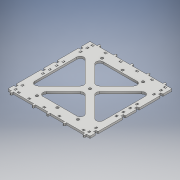
# Autodesk Inventor part: turtlebot_installation_side
Saved by Autodesk Inventor 2018 (Build 220112000, 112)
## iProperties
Created: 2018-07-15
Part Number: turtlebot_installation_side
Material: Generic
Document SubType Name: Modeling
Designer: Tsche
Density: 1 g/cm^3
Appearance: Default
Author: Tsche
Autodesk Inventor part; units mm, degrees
ref_plane "YZ Plane" through (0, 0, 0) normal (1, 0, 0) x (0, 1, 0)
ref_plane "XZ Plane" through (0, 0, 0) normal (0, 1, 0) x (-1, 0, 0)
ref_plane "XY Plane" through (0, 0, 0) normal (0, 0, 1) x (1, 0, 0)
sketch "Sketch1" plane through (0, 0, 0) normal (0, 0, 1) x (1, 0, 0)
  line L0 (-60, 60) -> (-49.5, 60)
  line L1 (60, 60) -> (60, 46.6)
  line L2 (60, -60) -> (55, -60)
  line L3 (-60, -60) -> (-60, -51.6)
  line L4 (-60, 60) -> (60, -60) construction
  line L5 (60, 60) -> (-60, -60) construction
  line L6 (-52, -60) -> (-52, -63)
  line L7 (-52, -63) -> (-55, -63)
  line L8 (-55, -63) -> (-55, -60)
  line L9 (-19.5, -60) -> (-19.5, -63)
  line L10 (-19.5, -63) -> (-22.5, -63)
  line L11 (-22.5, -63) -> (-22.5, -60)
  line L12 (-55, -60) -> (-60, -60)
  line L13 (-52, -60) -> (-55, -60) construction
  line L14 (-22.5, -60) -> (-52, -60)
  line L15 (-19.5, -60) -> (-22.5, -60) construction
  line L16 (-1.5, -60) -> (-19.5, -60)
  line L17 (22.75, -60) -> (1.5, -60)
  line L18 (52, -60) -> (25.75, -60)
  line L19 (-21, -63) -> (-21, -60) construction
  line L20 (-53.5, -60) -> (-53.5, -63) construction
  line L21 (-49, -55.7) -> (-46, -55.7)
  line L22 (-46, -55.7) -> (-46, -57)
  line L23 (-46, -57) -> (-49, -57)
  line L24 (-49, -57) -> (-49, -55.7)
  line L25 (-47.5, -57) -> (-47.5, -55.7) construction
  line L26 (-33.5, -55.7) -> (-30.5, -55.7)
  line L27 (-30.5, -55.7) -> (-30.5, -57)
  line L28 (-30.5, -57) -> (-33.5, -57)
  line L29 (-33.5, -57) -> (-33.5, -55.7)
  line L30 (-32, -57) -> (-32, -55.7) construction
  line L31 (0, -7.0711) -> (-36.9289, -44)
  line L32 (36.9289, -44) -> (0, -7.0711)
  line L33 (-84, 0) -> (84, 0) construction
  line L34 (0, 7.0711) -> (-36.9289, 44)
  line L35 (36.9289, 44) -> (0, 7.0711)
  line L36 (-7.0711, 0) -> (-50, -42.9289)
  line L37 (-50, -42.9289) -> (-50, 42.9289)
  line L38 (-50, 42.9289) -> (-7.0711, 0)
  line L39 (7.0711, 0) -> (50, -42.9289)
  line L40 (50, -42.9289) -> (50, 42.9289)
  line L41 (50, 42.9289) -> (7.0711, 0)
  line L42 (-60, -48.4) -> (-60, -11.6)
  line L43 (-60, 11.6) -> (-60, 43.4)
  line L44 (60, -51.6) -> (60, -60)
  line L45 (60, 8.4) -> (60, -8.4)
  line L46 (-54, -43.5) -> (-52.7, -43.5)
  line L47 (-52.7, -43.5) -> (-52.7, -46.5)
  line L48 (-52.7, -46.5) -> (-54, -46.5)
  line L49 (-54, -46.5) -> (-54, -43.5)
  line L50 (-54, 6.5) -> (-52.7, 6.5)
  line L51 (-52.7, 6.5) -> (-52.7, 3.5)
  line L52 (-52.7, 3.5) -> (-54, 3.5)
  line L53 (-54, 3.5) -> (-54, 6.5)
  line L54 (-54, 16.5) -> (-52.7, 16.5)
  line L55 (-52.7, 16.5) -> (-52.7, 13.5)
  line L56 (-52.7, 13.5) -> (-54, 13.5)
  line L57 (-54, 13.5) -> (-54, 16.5)
  line L58 (52.7, 16.5) -> (54, 16.5)
  line L59 (54, 16.5) -> (54, 13.5)
  line L60 (54, 13.5) -> (52.7, 13.5)
  line L61 (52.7, 13.5) -> (52.7, 16.5)
  line L62 (52.7, 6.5) -> (54, 6.5)
  line L63 (54, 6.5) -> (54, 3.5)
  line L64 (54, 3.5) -> (52.7, 3.5)
  line L65 (52.7, 3.5) -> (52.7, 6.5)
  line L66 (52.7, -43.5) -> (54, -43.5)
  line L67 (54, -43.5) -> (54, -46.5)
  line L68 (54, -46.5) -> (52.7, -46.5)
  line L69 (52.7, -46.5) -> (52.7, -43.5)
  line L70 (-54, -45) -> (-52.7, -45) construction
  line L71 (-54, 5) -> (-52.7, 5) construction
  line L72 (-54, 15) -> (-52.7, 15) construction
  line L73 (52.7, 15) -> (54, 15) construction
  line L74 (52.7, 5) -> (54, 5) construction
  line L75 (52.7, -45) -> (54, -45) construction
  line L76 (0, 60) -> (0, -60) construction
  line L77 (0, 88.2) -> (0, -88.2) construction
  line L78 (-1.5, -60) -> (1.5, -60) construction
  line L79 (22.75, -60) -> (25.75, -60) construction
  line L80 (52, -60) -> (55, -60) construction
  line L81 (60, -51.6) -> (60, -48.4) construction
  line L82 (60, 11.6) -> (60, 8.4) construction
  line L83 (-60, 8.4) -> (-60, 11.6) construction
  line L84 (-60, -48.4) -> (-60, -51.6) construction
  line L85 (60, 11.6) -> (56.9, 11.6)
  line L86 (56.9, 11.6) -> (56.9, 8.4)
  line L87 (56.9, 8.4) -> (60, 8.4)
  line L88 (60, -48.4) -> (56.9, -48.4)
  line L89 (56.9, -48.4) -> (56.9, -51.6)
  line L90 (56.9, -51.6) -> (60, -51.6)
  line L91 (56.9, -50) -> (60, -50) construction
  line L92 (56.9, 10) -> (60, 10) construction
  line L93 (-60, -48.4) -> (-56.9, -48.4)
  line L94 (-56.9, -48.4) -> (-56.9, -51.6)
  line L95 (-56.9, -51.6) -> (-60, -51.6)
  line L96 (-60, -50) -> (-56.9, -50) construction
  line L97 (-60, 11.6) -> (-56.9, 11.6)
  line L98 (-56.9, 11.6) -> (-56.9, 8.4)
  line L99 (-56.9, 8.4) -> (-60, 8.4)
  line L100 (-60, 10) -> (-56.9, 10) construction
  line L101 (-1.5, -60) -> (-1.5, -63)
  line L102 (-1.5, -63) -> (1.5, -63)
  line L103 (1.5, -63) -> (1.5, -60)
  line L104 (22.75, -60) -> (22.75, -63)
  line L105 (22.75, -63) -> (25.75, -63)
  line L106 (25.75, -63) -> (25.75, -60)
  line L107 (52, -60) -> (52, -63)
  line L108 (52, -63) -> (55, -63)
  line L109 (55, -63) -> (55, -60)
  line L110 (53.5, -60) -> (53.5, -63) construction
  line L111 (24.25, -60) -> (24.25, -63) construction
  line L112 (-11.5, -55.7) -> (-8.5, -55.7)
  line L113 (-8.5, -55.7) -> (-8.5, -57)
  line L114 (-8.5, -57) -> (-11.5, -57)
  line L115 (-11.5, -57) -> (-11.5, -55.7)
  line L116 (-10, -55.7) -> (-10, -57) construction
  line L117 (10.625, -55.7) -> (13.625, -55.7)
  line L118 (13.625, -55.7) -> (13.625, -57)
  line L119 (13.625, -57) -> (10.625, -57)
  line L120 (10.625, -57) -> (10.625, -55.7)
  line L121 (12.125, -55.7) -> (12.125, -57) construction
  line L122 (46, -55.7) -> (49, -55.7)
  line L123 (49, -55.7) -> (49, -57)
  line L124 (49, -57) -> (46, -57)
  line L125 (46, -57) -> (46, -55.7)
  line L126 (47.5, -55.7) -> (47.5, -57) construction
  line L127 (-1.5, 60) -> (-1.5, 63)
  line L128 (-1.5, 63) -> (1.5, 63)
  line L129 (1.5, 63) -> (1.5, 60)
  line L130 (-1.5, 60) -> (1.5, 60) construction
  line L131 (1.5, 60) -> (22.5, 60)
  line L132 (-22.5, 60) -> (-22.5, 63)
  line L133 (-22.5, 63) -> (-25.5, 63)
  line L134 (-25.5, 63) -> (-25.5, 60)
  line L135 (-46.5, 60) -> (-46.5, 63)
  line L136 (-46.5, 63) -> (-49.5, 63)
  line L137 (-49.5, 63) -> (-49.5, 60)
  line L138 (22.5, 60) -> (22.5, 63)
  line L139 (22.5, 63) -> (25.5, 63)
  line L140 (25.5, 63) -> (25.5, 60)
  line L141 (46.5, 60) -> (46.5, 63)
  line L142 (46.5, 63) -> (49.5, 63)
  line L143 (49.5, 63) -> (49.5, 60)
  line L144 (-49.5, 60) -> (-46.5, 60) construction
  line L145 (-46.5, 60) -> (-25.5, 60)
  line L146 (-25.5, 60) -> (-22.5, 60) construction
  line L147 (-22.5, 60) -> (-1.5, 60)
  line L148 (22.5, 60) -> (25.5, 60) construction
  line L149 (25.5, 60) -> (46.5, 60)
  line L150 (46.5, 60) -> (49.5, 60) construction
  line L151 (49.5, 60) -> (60, 60)
  line L152 (-48, 63) -> (-48, 60) construction
  line L153 (-24, 63) -> (-24, 60) construction
  line L154 (24, 63) -> (24, 60) construction
  line L155 (48, 63) -> (48, 60) construction
  line L156 (-13.5, 57) -> (-10.5, 57)
  line L157 (-10.5, 57) -> (-10.5, 55.7)
  line L158 (-10.5, 55.7) -> (-13.5, 55.7)
  line L159 (-13.5, 55.7) -> (-13.5, 57)
  line L160 (-12, 57) -> (-12, 55.7) construction
  line L161 (-32.5, 57) -> (-32.5, 55.7)
  line L162 (-34, 57) -> (-34, 55.7) construction
  line L163 (-35.5, 57) -> (-32.5, 57)
  line L164 (-35.5, 55.7) -> (-35.5, 57)
  line L165 (-32.5, 55.7) -> (-35.5, 55.7)
  line L166 (-54.5, 55.7) -> (-54.5, 57)
  line L167 (-53, 57) -> (-53, 55.7) construction
  line L168 (-51.5, 57) -> (-51.5, 55.7)
  line L169 (-54.5, 57) -> (-51.5, 57)
  line L170 (-51.5, 55.7) -> (-54.5, 55.7)
  line L171 (13.5, 57) -> (10.5, 57)
  line L172 (10.5, 57) -> (10.5, 55.7)
  line L173 (10.5, 55.7) -> (13.5, 55.7)
  line L174 (13.5, 55.7) -> (13.5, 57)
  line L175 (12, 57) -> (12, 55.7) construction
  line L176 (32.5, 57) -> (32.5, 55.7)
  line L177 (34, 57) -> (34, 55.7) construction
  line L178 (35.5, 57) -> (32.5, 57)
  line L179 (35.5, 55.7) -> (35.5, 57)
  line L180 (32.5, 55.7) -> (35.5, 55.7)
  line L181 (54.5, 55.7) -> (54.5, 57)
  line L182 (53, 57) -> (53, 55.7) construction
  line L183 (51.5, 57) -> (51.5, 55.7)
  line L184 (54.5, 57) -> (51.5, 57)
  line L185 (51.5, 55.7) -> (54.5, 55.7)
  line L186 (-54, -56.5) -> (-52.7, -56.5)
  line L187 (-52.7, -56.5) -> (-52.7, -53.5)
  line L188 (-52.7, -53.5) -> (-54, -53.5)
  line L189 (-54, -53.5) -> (-54, -56.5)
  line L190 (-54, -55) -> (-52.7, -55) construction
  line L191 (52.7, -56.5) -> (54, -56.5)
  line L192 (54, -56.5) -> (54, -53.5)
  line L193 (54, -53.5) -> (52.7, -53.5)
  line L194 (52.7, -53.5) -> (52.7, -56.5)
  line L195 (52.7, -55) -> (54, -55) construction
  line L196 (-60, -8.4) -> (-56.9, -8.4)
  line L197 (-56.9, -8.4) -> (-56.9, -11.6)
  line L198 (-56.9, -11.6) -> (-60, -11.6)
  line L199 (-60, -8.4) -> (-60, 8.4)
  line L200 (-60, -11.6) -> (-60, -8.4) construction
  line L201 (-60, -10) -> (-56.9, -10) construction
  line L202 (-54, -3.5) -> (-52.7, -3.5)
  line L203 (-52.7, -3.5) -> (-52.7, -6.5)
  line L204 (-52.7, -6.5) -> (-54, -6.5)
  line L205 (-54, -6.5) -> (-54, -3.5)
  line L206 (-54, -5) -> (-52.7, -5) construction
  line L207 (-54, -16.5) -> (-52.7, -16.5)
  line L208 (-52.7, -16.5) -> (-52.7, -13.5)
  line L209 (-52.7, -13.5) -> (-54, -13.5)
  line L210 (-54, -13.5) -> (-54, -16.5)
  line L211 (-54, -15) -> (-52.7, -15) construction
  line L212 (60, -8.4) -> (56.9, -8.4)
  line L213 (56.9, -8.4) -> (56.9, -11.6)
  line L214 (56.9, -11.6) -> (60, -11.6)
  line L215 (60, -8.4) -> (60, -11.6) construction
  line L216 (60, -10) -> (56.9, -10) construction
  line L217 (60, -11.6) -> (60, -48.4)
  line L218 (54, -3.5) -> (52.7, -3.5)
  line L219 (52.7, -3.5) -> (52.7, -6.5)
  line L220 (52.7, -6.5) -> (54, -6.5)
  line L221 (54, -6.5) -> (54, -3.5)
  line L222 (54, -5) -> (52.7, -5) construction
  line L223 (54, -15) -> (52.7, -15) construction
  line L224 (54, -16.5) -> (52.7, -16.5)
  line L225 (52.7, -16.5) -> (52.7, -13.5)
  line L226 (54, -13.5) -> (54, -16.5)
  line L227 (52.7, -13.5) -> (54, -13.5)
  line L228 (-60, 46.6) -> (-56.9, 46.6)
  line L229 (-56.9, 46.6) -> (-56.9, 43.4)
  line L230 (-56.9, 43.4) -> (-60, 43.4)
  line L231 (-60, 46.6) -> (-60, 60)
  line L232 (-60, 43.4) -> (-60, 46.6) construction
  line L233 (-60, 45) -> (-56.9, 45) construction
  line L234 (-54, 41.5) -> (-52.7, 41.5)
  line L235 (-52.7, 41.5) -> (-52.7, 38.5)
  line L236 (-52.7, 38.5) -> (-54, 38.5)
  line L237 (-54, 38.5) -> (-54, 41.5)
  line L238 (-54, 40) -> (-52.7, 40) construction
  line L239 (-54, 48.5) -> (-52.7, 48.5)
  line L240 (-52.7, 48.5) -> (-52.7, 51.5)
  line L241 (-52.7, 51.5) -> (-54, 51.5)
  line L242 (-54, 51.5) -> (-54, 48.5)
  line L243 (-54, 50) -> (-52.7, 50) construction
  line L244 (60, 46.6) -> (56.9, 46.6)
  line L245 (56.9, 46.6) -> (56.9, 43.4)
  line L246 (56.9, 43.4) -> (60, 43.4)
  line L247 (60, 46.6) -> (60, 43.4) construction
  line L248 (60, 43.4) -> (60, 11.6)
  line L249 (56.9, 45) -> (60, 45) construction
  line L250 (54, 41.5) -> (52.7, 41.5)
  line L251 (52.7, 41.5) -> (52.7, 38.5)
  line L252 (52.7, 38.5) -> (54, 38.5)
  line L253 (54, 38.5) -> (54, 41.5)
  line L254 (54, 40) -> (52.7, 40) construction
  line L255 (54, 48.5) -> (52.7, 48.5)
  line L256 (54, 50) -> (52.7, 50) construction
  line L257 (54, 51.5) -> (54, 48.5)
  line L258 (52.7, 51.5) -> (54, 51.5)
  line L259 (52.7, 48.5) -> (52.7, 51.5)
  circle A0 centre (0, 47.625) radius 1.85
  circle A1 centre (0, -47.625) radius 1.85
  line L260 (36.9289, -44) -> (-36.9289, -44)
  line L261 (36.9289, 44) -> (-36.9289, 44)
  circle A2 centre (30, -47.625) radius 1.85
  circle A3 centre (-30, -47.625) radius 1.85
  circle A4 centre (30, 47.625) radius 1.85
  circle A5 centre (-30, 47.625) radius 1.85
  circle A6 centre (0, 0) radius 1.85
  point P0 (0, 0)
  point P1 (0, 0)
  point P2 (0, -63)
  point P3 (0, 63)
  point P4 (-31, 50)
  dimension "d0" = 120
  dimension "d1" = 120
  dimension "d2" = 3
  dimension "d3" = 3
  dimension "d12" = 3
  dimension "d13" = 3
  dimension "d15" = 6.5
  dimension "d19" = 32.5
  dimension "d20" = 3
  dimension "d21" = 1.3
  dimension "d28" = 6
  dimension "d30" = 3
  dimension "d31" = 1.3
  dimension "d32" = 11
  dimension "d35" = 3
  dimension "d36" = 10
  dimension "d37" = 5
  dimension "d38" = 5
  dimension "d51" = 3
  dimension "d52" = 1.3
  dimension "d53" = 3
  dimension "d54" = 3
  dimension "d55" = 1.3
  dimension "d56" = 1.3
  dimension "d57" = 3
  dimension "d58" = 1.3
  dimension "d59" = 3
  dimension "d60" = 3
  dimension "d61" = 1.3
  dimension "d85" = 60
  dimension "d86" = 10
  dimension "d87" = 3.2
  dimension "d88" = 3.2
  dimension "d90" = 3.1
  dimension "d92" = 3.1
  dimension "d93" = 3.2
  dimension "d94" = 10
  dimension "d95" = 3.1
  dimension "d96" = 3.2
  dimension "d97" = 60
  dimension "d98" = 5
  dimension "d99" = 6
  dimension "d100" = 5
  dimension "d101" = 6
  dimension "d102" = 5
  dimension "d103" = 5
  dimension "d104" = 6
  dimension "d105" = 5
  dimension "d106" = 3
  dimension "d107" = 3
  dimension "d108" = 3
  dimension "d109" = 6.5
  dimension "d110" = 24.25
  dimension "d111" = 3
  dimension "d112" = 1.3
  dimension "d113" = 3
  dimension "d114" = 1.3
  dimension "d115" = 3
  dimension "d116" = 1.3
  dimension "d117" = 12.125
  dimension "d118" = 6
  dimension "d119" = 11
  dimension "d122" = 3
  dimension "d123" = 3
  constraints: 520 end point, 174 parallel, 167 perpendicular, 76 symmetric about line, 69 midpoint, 41 point on line, 38 horizontal, 19 collinear, 13 equal length, 7 centre point, 7 vertical, 1 coincident, 1 equal radius, 29 other
  measures "d0" distance of L2.start L3.start
  measures "d1" distance of L1.start L2.start
  measures "d2" distance of L6.end L7.end
  measures "d3" distance of L6.start L6.end
  measures "d12" distance of L9.end L10.end
  measures "d13" distance of L9.start L9.end
  measures "d15" distance between parallel lines of L3 L20
  measures "d19" distance between parallel lines of L19 L20
  measures "d20" distance of L21.start L21.end
  measures "d21" distance of L23.end L21.start
  measures "d28" distance between parallel lines of L20 L25
  measures "d30" distance of L29.end L27.start
  measures "d31" distance of L29.start L29.end
  measures "d32" distance between parallel lines of L30 L19
  measures "d35" distance between parallel lines of L23 L14
  measures "d36" distance between parallel lines of L3 L37
  measures "d37" distance between parallel lines of L36 L5
  measures "d38" distance between parallel lines of L31 L5
  measures "d51" distance of L46.end L47.end
  measures "d52" distance of L47.end L48.end
  measures "d53" distance of L50.end L51.end
  measures "d54" distance of L54.end L55.end
  measures "d55" distance of L54.start L54.end
  measures "d56" distance of L58.start L58.end
  measures "d57" distance of L60.end L58.start
  measures "d58" distance of L63.end L64.end
  measures "d59" distance of L64.end L62.start
  measures "d60" distance of L68.end L66.start
  measures "d61" distance of L66.start L66.end
  measures "d85" distance between parallel lines of L92 L91
  measures "d86" distance between parallel lines of L2 L91
  measures "d87" distance of L85.end L86.end
  measures "d88" distance of L88.end L89.end
  measures "d90" distance of L86.end L45.start
  measures "d92" distance of L94.end L3.end
  measures "d93" distance of L93.end L94.end
  measures "d94" distance between parallel lines of L12 L96
  measures "d95" distance of L98.end L83.start
  measures "d96" distance of L97.end L98.end
  measures "d97" distance between parallel lines of L96 L100
  measures "d98" distance between parallel lines of L70 L96
  measures "d99" distance between parallel lines of L42 L49
  measures "d100" distance between parallel lines of L100 L71
  measures "d101" distance between parallel lines of L42 L53
  measures "d102" distance between parallel lines of L100 L72
  measures "d103" distance between parallel lines of L92 L73
  measures "d104" distance between parallel lines of L45 L63
  measures "d105" distance between parallel lines of L91 L75
  measures "d106" distance of L101.end L102.end
  measures "d107" distance of L104.end L105.end
  measures "d108" distance of L107.end L108.end
  measures "d109" distance between parallel lines of L44 L110
  measures "d110" distance between parallel lines of L77 L111
  measures "d111" distance of L113.end L114.end
  measures "d112" distance of L114.end L112.start
  measures "d113" distance of L119.start L120.start
  measures "d114" distance of L120.start L120.end
  measures "d115" distance of L124.start L125.start
  measures "d116" distance of L125.start L125.end
  measures "d117" distance between parallel lines of L77 L121
  measures "d118" distance between parallel lines of L110 L126
  measures "d119" distance between parallel lines of L19 L116
  measures "d122" distance of L127.end L128.end
  measures "d123" distance of L127.start L127.end
extrude "Extrusion2" add sketch "Sketch1" along normal blind 3
fillet "Fillet1" radius 1 40 edges at (-60, 11.6, 1.5) (-60, 8.4, 1.5) (-60, -60, 1.5) (-60, -51.6, 1.5) (-60, -48.4, 1.5) (-55, -63, 1.5) (-52, -63, 1.5) (-22.5, -63, 1.5) (-19.5, -63, 1.5) (-1.5, -63, 1.5) (1.5, -63, 1.5) (22.75, -63, 1.5) (25.75, -63, 1.5) (52, -63, 1.5) (55, -63, 1.5) (60, -60, 1.5) (60, -51.6, 1.5) (60, -48.4, 1.5) (60, 8.4, 1.5) (60, 11.6, 1.5) (-49.5, 63, 1.5) (-46.5, 63, 1.5) (-60, 60, 1.5) (-25.5, 63, 1.5) (-22.5, 63, 1.5) (-1.5, 63, 1.5) (1.5, 63, 1.5) (22.5, 63, 1.5) (25.5, 63, 1.5) (46.5, 63, 1.5) (49.5, 63, 1.5) (60, 60, 1.5) (-60, -11.6, 1.5) (-60, -8.4, 1.5) (60, -11.6, 1.5) (60, -8.4, 1.5) (-60, 43.4, 1.5) (-60, 46.6, 1.5) (60, 43.4, 1.5) (60, 46.6, 1.5)
chamfer "Chamfer1" distance 1 angle 45 54 edges at (-54, 15, 3) (-54, 15, 0) (-54, 5, 3) (-54, 5, 0) (-54, -45, 3) (-54, -45, 0) (-47.5, -57, 3) (-47.5, -57, 0) (-32, -57, 3) (-32, -57, 0) (-10, -57, 3) (-10, -57, 0) (12.125, -57, 3) (12.125, -57, 0) (47.5, -57, 3) (47.5, -57, 0) (54, -45, 3) (54, -45, 0) (54, 5, 3) (54, 5, 0) (54, 15, 3) (54, 15, 0) (-53, 57, 3) (-53, 57, 0) (-34, 57, 3) (-34, 57, 0) (-12, 57, 3) (-12, 57, 0) (12, 57, 3) (12, 57, 0) (34, 57, 3) (34, 57, 0) (53, 57, 3) (53, 57, 0) (-54, -55, 3) (-54, -55, 0) (54, -55, 0) (54, -55, 3) (-54, -5, 3) (-54, -15, 3) (-54, -5, 0) (-54, -15, 0) (54, -15, 3) (54, -15, 0) (54, -5, 3) (54, -5, 0) (54, 40, 0) (54, 40, 3) (54, 50, 0) (54, 50, 3) (-54, 40, 3) (-54, 40, 0) (-54, 50, 0) (-54, 50, 3)
fillet "Fillet2" radius 5 12 edges at (-50, 42.9289, 1.5) (-36.9289, 44, 1.5) (36.9289, 44, 1.5) (0, 7.0711, 1.5) (-7.0711, 0, 1.5) (7.0711, 0, 1.5) (0, -7.0711, 1.5) (-50, -42.9289, 1.5) (-36.9289, -44, 1.5) (36.9289, -44, 1.5) (50, -42.9289, 1.5) (50, 42.9289, 1.5)
body "Solid1"
body "Solid2"
